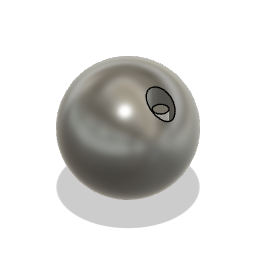
ball v4 (Autodesk Fusion 360 design; units mm, degrees)
Autodesk Fusion 360 part; units mm, degrees
sphere "球体基本要素2" add diameter 25 placed x (0, 0, -1) y (0, 1, 0) z (1, 0, 0) at (0, 27.5, 0)
ref_plane "工作平面1" through (0, 27.5, 0) normal (0, 1, 0) x (0, 0, 1)
sketch "草图6" plane through (0, 27.5, 0) normal (0, 1, 0) x (1, 0, 0)
  circle A0 centre (8, 0) radius 1.5
  circle A1 centre (8, 0) radius 2.5
  dimension "d25" = 3
  dimension "d26" = 5
  dimension "d27" = 8
  constraint concentric A0 A1
  constraint horizontal origin A0.centre
  measures "d25" diameter of A0
  measures "d26" diameter of A1
  measures "d27" distance of origin A0.centre
extrude "拉伸6" cut sketch "草图6" along normal through all
extrude "拉伸7" cut sketch "草图6" along normal blind 16 contours A0
extrude "拉伸8" add sketch "草图6" along normal blind 8 contours A0
thread "螺纹3" "ISO Metric profile 3.0 M3x0.5 6g" major diameter 2.927 minor diameter 2.3555 pitch 0.5 angle 60 resizes the face on face at (9.4925, 30.1667, 0.1494)
sketch "草图7" plane through (0, 0, 0) normal (0, 0, 1) x (1, 0, 0)
  line L0 (-0.0753, 40.4285) -> (-0.0753, 14.5)
  line L1 (-0.0753, 14.5) -> (-0.0753, 40.5)
  line L2 (-0.0753, 40.5) -> (-0.0753, 14.5)
  dimension "d33" = 26
  constraint vertical L0
  constraint parallel L0 L1
  constraint parallel L1 L2
  measures "d33" distance of L1.end L0.end
